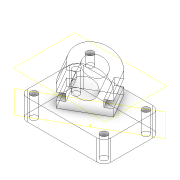
# Autodesk Inventor part: Chpt9_Tutorial
Saved by Autodesk Inventor 2017 (Build 210142000, 142)
## iProperties
Created: 2018-11-02
Part Number: Chpt9_Tutorial
Material: Generic
Document SubType Name: Modeling
Designer: jpb34
Density: 1 g/cm^3
Appearance: Default
Author: jpb34
Autodesk Inventor part; units mm, degrees
sketch "Sketch1" plane through (0, 0, 0) normal (0, 1, 0) x (-1, 0, 0)
  line L0 (31.75, 25.4) -> (-31.75, 25.4)
  line L1 (-38.1, 19.05) -> (-38.1, -19.05)
  line L2 (-31.75, -25.4) -> (31.75, -25.4)
  line L3 (38.1, -19.05) -> (38.1, 19.05)
  arc A0 (31.75, -25.4) -> (38.1, -19.05) centre (31.75, -19.05) ccw
  arc A1 (38.1, 19.05) -> (31.75, 25.4) centre (31.75, 19.05) ccw
  arc A2 (-31.75, 25.4) -> (-38.1, 19.05) centre (-31.75, 19.05) ccw
  arc A3 (-38.1, -19.05) -> (-31.75, -25.4) centre (-31.75, -19.05) ccw
  circle A4 centre (31.75, -19.05) radius 3.175
  circle A5 centre (31.75, 19.05) radius 3.175
  circle A6 centre (-31.75, 19.05) radius 3.175
  circle A7 centre (-31.75, -19.05) radius 3.175
  point P0 (0, 0)
  dimension "d0" = 6.35
  dimension "d1" = 50.8
  dimension "d2" = 76.2
  dimension "d3" = 38.1
  dimension "d4" = 25.4
  dimension "d5" = 6.35
  dimension "d6" = 6.35
  dimension "d7" = 6.35
  dimension "d8" = 6.35
  constraints: 8 centre point, 8 end point, 8 point on circle, 8 tangent, 4 coincident, 3 equal radius, 2 parallel, 1 horizontal, 1 perpendicular
  measures "d0" radius of A0
  measures "d1" distance between parallel lines of L2 L0
  measures "d2" distance between parallel lines of L1 L3
  measures "d3" distance from line of point (0, 0) L1
  measures "d4" distance from line of point (0, 0) L0
  measures "d5" diameter of A4
  measures "d6" diameter of A5
  measures "d7" diameter of A6
  measures "d8" diameter of A7
extrude "Extrusion1" add sketch "Sketch1" along normal blind 19.05
ref_plane "Work Plane1" through (0, 0, 0) normal (0.5, 0, 0.866) x (0, 1, 0)
sketch "Sketch2" plane through (0, 0, 0) normal (0.5, 0, 0.866) x (0, 1, 0)
  line L0 (19.05, -40.1963) -> (19.05, 14.7963) projected
  line L1 (0, 14.7963) -> (19.05, 14.7963) projected
  line L2 (25.3995, 19.0504) -> (25.3995, 12.7004)
  line L3 (25.3995, 12.7004) -> (31.7495, 12.7005)
  line L4 (31.7495, 12.7005) -> (31.7495, 19.0505)
  line L5 (31.7495, 19.0505) -> (38.0995, 19.0505)
  line L6 (38.1, -19.0495) -> (31.75, -19.0495)
  line L7 (31.75, -19.0495) -> (31.7499, -12.6995)
  line L8 (31.7499, -12.6995) -> (25.3999, -12.6996)
  line L9 (25.3999, -12.6996) -> (25.4, -19.0496)
  line L10 (19.05, -19.0497) -> (25.4, -19.0496)
  arc A0 (38.1, -19.0495) -> (38.0995, 19.0505) centre (38.1, 0.0005) ccw
  circle A1 centre (38.1, 0.0005) radius 9.525
  line L11 (25.3995, 19.0504) -> (19.05, 19.0504)
  line L12 (19.05, 19.0504) -> (19.05, -19.0497)
  point P0 (0, 0)
  dimension "d19" = 38.1
  dimension "d20" = 19.05
  dimension "d21" = 6.35
  dimension "d22" = 6.35
  dimension "d23" = 6.35
  dimension "d25" = 6.35
  dimension "d28" = 19.05
  dimension "d29" = 19.05
  dimension "d30" = 6.35
  dimension "d31" = 6.3495
  dimension "d32" = 38.1001
  constraints: 22 end point, 7 point on line, 5 perpendicular, 2 centre point, 2 point on circle, 1 coincident, 1 collinear, 1 horizontal
  measures "d19" distance of L5.end L6.start
  measures "d20" distance from line of point (0, 0) L6
  measures "d21" distance of L6.end L7.end
  measures "d22" distance of L7.end L8.end
  measures "d23" distance of L10.start L9.end
  measures "d25" distance of L3.end L4.end
  measures "d28" diameter of A1
  measures "d29" distance from line of L0 A0.centre
  measures "d30" distance of L2.start L2.end
  measures "d31" distance of L2.start L11.end
  measures "d32" distance of L11.end L10.start
extrude "Extrusion2" add sketch "Sketch2" along normal mid plane 25.4
ref_plane "Work Plane2" through (0, 38.1, 0) normal (0, 1, 0) x (1, 0, 0)
sketch "Sketch3" plane through (0, 38.1, 0) normal (0, 1, 0) x (1, 0, 0)
  circle A0 centre (0, 0) radius 3.175
  dimension "d36" = 6.35
  constraints: 1 centre point, 1 coincident
  measures "d36" diameter of A0
extrude "Extrusion3" cut sketch "Sketch3" along normal blind 25.4
equation "\"d6\" = d5"
equation "\"d7\" = d5"
equation "\"d8\" = d5"
body "Solid1"
